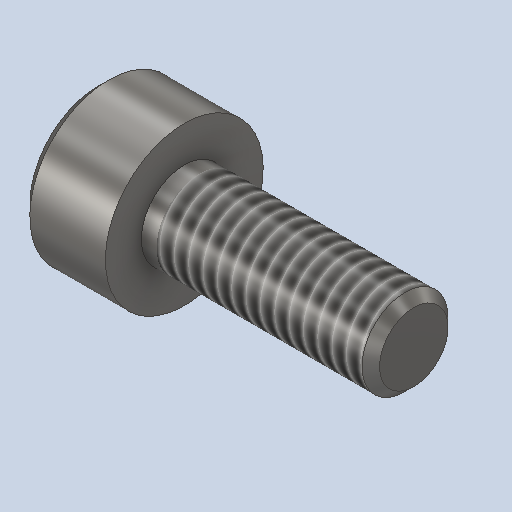
# Autodesk Inventor part: BOX-CBF3-8
Saved by Autodesk Inventor 2022 (Build 260153000, 153)
## iProperties
Created: 2022-11-06
Part Number: BOX-CBF3-8
Material: ステンレス鋼
Catalog Web Link: www.cadenas.de
Description: BOX-CBF-(Box Set) Hexagon Socket Cap Screws
Vendor: MISUMI
Document SubType Name: Modeling
Designer: psAdmin
Manufacturer: MISUMI
Mass: 0.941658 g
Surface Area: 1.82198 cm^2
Volume: 0.117707 cm^3
Density: 8 g/cm^3
Appearance: 半つや出し
Category: PARTsolutions
Company: MISUMI
PSOL_IDENT_0: {$CADENAS_DATA/23d-libs/misumi/metric/27_screws_nuts/box_cbf.prj},163 {VTYP=3D},{NB=BOX-CBF3-8},{LIN
PSOL_IDENT_1: A=BOX-CBF3-8},{NN=BOX-CBF},{DATE=30.06.2021 13:09:20},{GEOMDATE=25.03.2010 00:00:00},{VERSION=},{LIN
PSOL_IDENT_2: EID=40},{WBVAR=L},{WBNUMERIC=L}  {NB=BOX-CBF3-8},{LINA=BOX-CBF3-8},{KT=DUMMY},{PN=BOX-CBF3-8},{TYPE=
PSOL_IDENT_3: BOX-CBF},{MAT=4137 Alloy Steel},{ST=Black Oxide},{HARD=38~43HRC},{SC=12.9},{M1=3},{M=3.0},{L=8},{L0=
PSOL_IDENT_4: 5,6,8,10,12,15,20,25,30},{LL=Full Thread Screws},{LL0=8},{MP=3x0.5},{PITCH=0.50},{A=5.5},{E=3.0},{B=
PSOL_IDENT_5: 2.5},{PCS=1,000 pcs./box}
NB: BOX-CBF3-8
NN: BOX-CBF
NT: (Box Set) Hexagon Socket Cap Screws
NBSYN: $PN.
LINA: BOX-CBF3-8
CATALOG: Misumi
PN: BOX-CBF3-8
MAT: 4137 Alloy Steel
ST: Black Oxide
HARD: 38~43HRC
SC: 12.9
M1: 3
L: 8
LL: Full Thread Screws
MP: 3x0.5
PITCH: 0.5
A: 5.5
E: 3
B: 2.5
PCS: 1,000 pcs./box
SUPPLIER: MISUMI
ARTICLENO: BOX-CBF3-8
BOMINFO: BOX-CBF3-8
CREATOR: CADENAS GmbH
Title: BOX-CBF3-8
Author: Cadenas PARTsolutions
Comments: (Box Set) Hexagon Socket Cap Screws
Autodesk Inventor part; units mm, degrees
ref_plane "YZ Plane" through (0, 0, 0) normal (1, 0, 0) x (0, 1, 0)
ref_plane "XZ Plane" through (0, 0, 0) normal (0, 1, 0) x (-1, 0, 0)
ref_plane "XY Plane" through (0, 0, 0) normal (0, 0, 1) x (1, 0, 0)
sketch "Sketch_1" plane through (0, 0, 0) normal (0, 0, 1) x (1, 0, 0)
  line L0 (8, 0) -> (-1.1807, 0)
  line L1 (-1.1807, 0) -> (-1.5156, 1.25)
  line L2 (-1.5156, 1.25) -> (-3, 1.25)
  line L3 (-3, 1.25) -> (-3, 2.3833)
  line L4 (-3, 2.3833) -> (-2.6333, 2.75)
  line L5 (-2.6333, 2.75) -> (0, 2.75)
  line L6 (0, 2.75) -> (0, 1.5)
  line L7 (0, 1.5) -> (7.6935, 1.5)
  line L8 (7.6935, 1.5) -> (8, 1.1935)
  line L9 (8, 1.1935) -> (8, 0)
  line L10 (8, 0) -> (-1.1807, 0)
  constraints: 22 end point
revolve "Revolution1" add sketch "Sketch_1" angle 360 about axis through (8, 0, 0) along (1, 0, 0)
thread "Thread1" size "M3x0.5" class "6g" standard "ISO Metric profile" length 7.1626
sketch "Sketch_2" plane through (-3, 0, 0) normal (1, 0, 0) x (0, 0, -1)
  line L0 (-1.25, -0.7217) -> (0, -1.4434)
  line L1 (0, -1.4434) -> (1.25, -0.7217)
  line L2 (1.25, -0.7217) -> (1.25, 0.7217)
  line L3 (1.25, 0.7217) -> (0, 1.4434)
  line L4 (0, 1.4434) -> (-1.25, 0.7217)
  line L5 (-1.25, 0.7217) -> (-1.25, -0.7217)
  constraints: 12 end point
extrude "Extrusion1" cut sketch "Sketch_2" along normal blind 1.5
body "Solid1"
